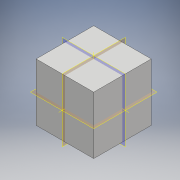
# Autodesk Inventor part: Rubik's Cube
Saved by Autodesk Inventor 2017 (Build 210142000, 142)
## iProperties
Created: 2018-12-03
Part Number: Rubik's Cube
Material: Generic
Document SubType Name: Modeling
Designer: Eric the Great
Density: 1 g/cm^3
Appearance: Default
Author: Eric the Great
Autodesk Inventor part; units mm, degrees
ref_plane "YZ Plane" through (0, 0, 0) normal (1, 0, 0) x (0, 1, 0)
ref_plane "XZ Plane" through (0, 0, 0) normal (0, 1, 0) x (-1, 0, 0)
ref_plane "XY Plane" through (0, 0, 0) normal (0, 0, 1) x (1, 0, 0)
sketch "Sketch1" plane through (0, 0, 0) normal (0, 1, 0) x (-1, 0, 0)
  line L0 (-27.94, 27.94) -> (27.94, 27.94)
  line L1 (27.94, 27.94) -> (27.94, -27.94)
  line L2 (27.94, -27.94) -> (-27.94, -27.94)
  line L3 (-27.94, -27.94) -> (-27.94, 27.94)
  line L4 (-27.94, 27.94) -> (27.94, -27.94) construction
  line L5 (27.94, 27.94) -> (-27.94, -27.94) construction
  point P0 (0, 0)
  dimension "d0" = 55.88
  dimension "d1" = 55.88
  constraints: 12 end point, 2 midpoint, 2 parallel, 1 horizontal, 1 perpendicular
  measures "d0" distance of L1.end L2.end
  measures "d1" distance of L0.end L1.end
extrude "Extrusion1" add sketch "Sketch1" along normal blind 55.88
ref_plane "Work Plane1" through (0, 0, 27.94) normal (1, 0, 0) x (0, 0, -1)
ref_plane "Work Plane2" through (-27.94, 0, 0) normal (0, 0, 1) x (1, 0, 0)
ref_plane "Work Plane3" through (0, 27.94, 0) normal (0, 1, 0) x (1, 0, 0)
body "Solid1"
